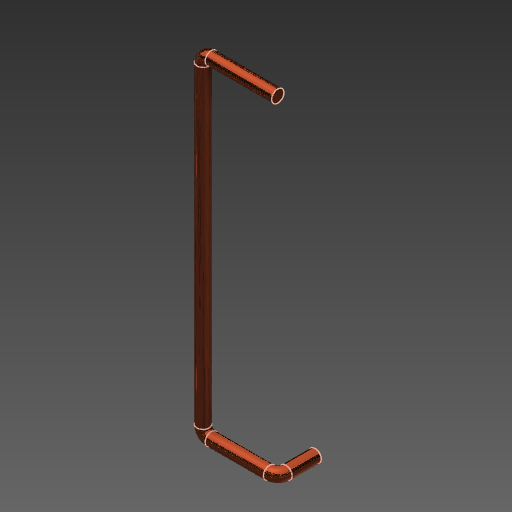
# Autodesk Inventor part: TopPipe
Saved by Autodesk Inventor 2020.4 (Build 244396010, 396A)
## iProperties
Created: 2022-09-12
Part Number: TopPipe
Material: Copper, Cast
Document SubType Name: Modeling
Designer: Val
Density: 8.94 g/cm^3
Appearance: Copper - Satin
Author: Val
Autodesk Inventor part; units mm, degrees
ref_plane "YZ Plane" through (0, 0, 0) normal (1, 0, 0) x (0, 1, 0)
ref_plane "XZ Plane" through (0, 0, 0) normal (0, 1, 0) x (-1, 0, 0)
sketch "PipeSide" plane through (0, 0, 0) normal (0, 0, 1) x (1, 0, 0)
  line L0 (-76.2, 336.55) -> (-76.2, 0) construction
  line L1 (-76.2, 0) -> (0, 0) construction
  line L2 (-76.2, 336.55) -> (0, 336.55) construction
  ellipse E0 centre (0, 0) end of major axis (0, 6.35) minor radius 5.4993 construction
  point P0 (75.9666, 233.9144)
  point P1 (76.9893, 233.9144)
  dimension "d1" = 76.2
  dimension "d2" = 336.55
  dimension "d3" = 76.2
  constraints: 6 end point, 2 coincident, 2 perpendicular, 1 centre point, 1 vertical
  measures "d1" distance of L0.start L2.end
  measures "d2" distance of L0.start L0.end
  measures "d3" distance of L0.end L1.end
sketch "PipeProfile" plane through (0, 0, 38.1) normal (0, 0, 1) x (1, 0, 0)
  circle A0 centre (0, 0) radius 6.35
  dimension "d5" = 12.7
  constraints: 1 centre point, 1 coincident
  measures "d5" diameter of A0
sketch3d "Pipe3D"
  line L0 (0, 0, 38.1) -> (0, 0, 8.382)
  arc A0 (0, 0, 8.382) -> (-8.382, 0, 0) centre (-8.382, 0, 8.382) ccw
  line L1 (-8.382, 0, 0) -> (-67.818, 0, 0)
  arc A1 (-67.818, 0, 0) -> (-76.2, 8.382, 0) centre (-67.818, 8.382, 0) ccw
  line L2 (-76.2, 8.382, 0) -> (-76.2, 328.168, 0)
  arc A2 (-76.2, 328.168, 0) -> (-67.818, 336.55, 0) centre (-67.818, 328.168, 0) ccw
  line L3 (-67.818, 336.55, 0) -> (0, 336.55, 0)
  dimension "d4" = 38.1
  dimension "d13" = 8.382
  dimension "d14" = 8.382
  dimension "d15" = 8.382
sweep "PipeFeature" add profiles "PipeProfile" path "Pipe3D"
mirror "MirrorFeature" about plane through (0, 0, 0) normal (0, 0, 1) remove original yes
ref_plane "TubeProfilePlane" through (0, 0, 38.1) normal (0, 0, 1) x (1, 0, 0)
equation "\"d14\" = d13"
equation "\"d15\" = d13"
body "Solid5"
